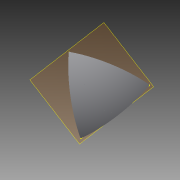
# Autodesk Inventor part: ommatid
Saved by Autodesk Inventor 2015 SP2 (Build 190223200, 223)
## iProperties
Created: 2015-05-04
Part Number: ommatid
Material: Generic
Document SubType Name: Modeling
Designer: foote
Density: 1 g/cm^3
Appearance: Default
Mass: 180.071 g
Surface Area: 758.025 cm^2
Volume: 180.071 cm^3
Author: foote
Autodesk Inventor part; units mm, degrees
note: some values were not read from the file. Chosen so that the rebuilt part matches the saved one: kept side of "Split8".
sketch "Sketch1" plane through (0, 0, 0) normal (0, 0, 1) x (1, 0, 0)
  line L0 (-46.99, -29.0414) -> (46.99, -29.0414)
  line L1 (46.99, -29.0414) -> (46.99, 29.0414)
  line L2 (46.99, 29.0414) -> (-46.99, 29.0414)
  line L3 (-46.99, 29.0414) -> (-46.99, -29.0414)
  point P0 (0, 0)
  dimension "d3" = 46.99
  dimension "d4" = 46.99
  dimension "d5" = 29.0414
  dimension "d6" = 29.0414
  constraints: 8 end point, 2 parallel, 1 horizontal, 1 perpendicular
  measures "d3" distance from line of point (0, 0) L3
  measures "d4" distance from line of L1 point (0, 0)
  measures "d5" distance from line of L0 point (0, 0)
  measures "d6" distance from line of L2 point (0, 0)
sketch "Sketch4" plane through (0, 0, 0) normal (1, 0, 0) x (0, 1, 0)
  line L0 (-47.0942, 0) -> (47.0942, 0)
  line L1 (-46.99, -29.0414) -> (46.99, -29.0414)
  line L2 (46.99, -29.0414) -> (46.99, 29.0414)
  line L3 (46.99, 29.0414) -> (-46.99, 29.0414)
  line L4 (-46.99, 29.0414) -> (-46.99, -29.0414)
  point P0 (0, 0)
  point P1 (0, 0)
  dimension "d38" = 29.0414
  dimension "d39" = 29.0414
  dimension "d40" = 46.99
  dimension "d41" = 46.99
  constraints: 10 end point, 2 parallel, 1 horizontal, 1 midpoint, 1 perpendicular
  measures "d38" distance from line of L3 point (0, 0)
  measures "d39" distance from line of L1 point (0, 0)
  measures "d40" distance from line of L2 point (0, 0)
  measures "d41" distance from line of L4 point (0, 0)
sketch "Sketch5" plane through (0, 0, 0) normal (0, 1, 0) x (-1, 0, 0)
  line L0 (-29.0414, -46.99) -> (29.0414, -46.99)
  line L1 (29.0414, -46.99) -> (29.0414, 46.99)
  line L2 (29.0414, 46.99) -> (-29.0414, 46.99)
  line L3 (-29.0414, 46.99) -> (-29.0414, -46.99)
  point P0 (0, 0)
  point P1 (0, 0)
  point P2 (0, 0)
  dimension "d31" = 29.0414
  dimension "d32" = 29.0414
  dimension "d33" = 46.99
  dimension "d34" = 46.99
  constraints: 8 end point, 2 parallel, 1 coincident, 1 horizontal, 1 perpendicular
  measures "d31" distance from line of point (0, 0) L3
  measures "d32" distance from line of L1 point (0, 0)
  measures "d33" distance from line of L0 point (0, 0)
  measures "d34" distance from line of L2 point (0, 0)
sketch3d "3D Sketch1"
ref_plane "Work Plane1" through (0, 46.99, 29.0414) normal (-0.5773503, -0.5773503, -0.5773503) x (0.809017, -0.309017, -0.5)
sketch "Sketch6" plane through (0, 46.99, 29.0414) normal (-0.5773503, -0.5773503, -0.5773503) x (0.809017, -0.309017, -0.5)
  line L0 (0, 0) -> (29.0414, 50.3012) projected
  line L1 (0, 0) -> (58.0828, 0) projected
  line L2 (29.0414, 50.3012) -> (58.0828, 0) projected
  line L3 (14.5207, 25.1506) -> (29.0414, 0)
  line L4 (29.0414, 0) -> (43.5621, 25.1506)
  line L5 (14.5207, 25.1506) -> (43.5621, 25.1506)
  circle A0 centre (29.0414, 16.7671) radius 12.7
  dimension "d48" = 25.4
  constraints: 6 end point, 3 midpoint, 1 centre point, 1 coincident, 1 horizontal
  measures "d48" diameter of A0
sketch3d "3D Sketch2"
ref_plane "Work Plane2" through (-6.7458, 40.2442, 22.2957) normal (-0.5773503, -0.5773503, -0.5773503) x (0.809017, -0.309017, -0.5)
sketch "Sketch8" plane through (-6.7458, 40.2442, 22.2957) normal (-0.5773503, -0.5773503, -0.5773503) x (0.809017, -0.309017, -0.5)
  line L0 (18.3857, 22.9192) -> (39.6971, 22.9192)
  line L1 (39.6971, 22.9192) -> (29.0414, 4.4629)
  line L2 (29.0414, 4.4629) -> (18.3857, 22.9192)
  line L3 (29.0414, 4.4629) -> (50.3529, 4.4629)
  line L4 (39.6971, 22.9192) -> (50.3529, 4.4629)
  line L5 (7.73, 4.4629) -> (18.3857, 22.9192)
  line L6 (7.73, 4.4629) -> (29.0414, 4.4629)
  line L7 (39.6971, 22.9192) -> (29.0414, 41.3754)
  line L8 (18.3857, 22.9192) -> (29.0414, 41.3754)
  point P0 (29.0414, 16.7671)
  constraints: 18 end point, 3 horizontal
ref_plane "Work Plane4" through (0, 46.99, 29.0414) normal (-0.809017, -0.309017, 0.5) x (0, -0.8506508, -0.5257311)
sketch "Sketch9" plane through (0, 46.99, 29.0414) normal (-0.809017, -0.309017, 0.5) x (0, -0.8506508, -0.5257311)
  line L0 (0, 0) -> (55.2401, 0) projected
  line L1 (55.2401, 0) -> (30.536, 49.4082) projected
  line L2 (0, 0) -> (14.7032, 0)
  line L3 (30.536, 49.4082) -> (37.1114, 36.2572)
  line L4 (55.2401, 0) -> (79.9442, 39.9721) construction
  arc A0 (30.536, 49.4082) -> (0, 0) centre (55.2401, 0) ccw
  dimension "d43" = 46.99
  constraints: 6 end point, 2 point on circle, 1 centre point, 1 coincident, 1 collinear, 1 horizontal
  measures "d43" distance of L0.end L4.end
ref_plane "Work Plane7" through (0, 46.99, 29.0414) normal (-0.309017, 0.5, -0.809017) x (0.809017, -0.309017, -0.5)
ref_plane "Work Plane9" through (46.99, 29.0414, 0) normal (-0.1624598, 0.2628656, 0.9510565) x (-0.8506508, -0.5257311, 0)
revolve "Revolution2" add sketch "Sketch9" angle 58.283 about axis through (0, 0, 0) along (-0.5, 0.809017, -0.309017)
ref_plane "Work Plane10" through (0, 0, 0) normal (0.5, -0.809017, -0.309017) x (0.8506508, 0.5257311, 0)
ref_plane "Work Plane11" through (0, 46.99, 29.0414) normal (-0.309017, 0.5, -0.809017) x (0.809017, -0.309017, -0.5)
split "Split4" plane through (0, 0, 0) removes the side toward (0.5, -0.809017, -0.309017)
split "Split5" plane through (0, 46.99, 29.0414) removes the side toward (-0.309017, 0.5, -0.809017)
ref_plane "Work Plane13" through (18.7929, 30.4076, 49.2006) normal (0, 0.8506508, -0.5257311) x (0.809017, -0.309017, -0.5)
ref_plane "Work Plane14" through (49.2006, 18.7929, 30.4076) normal (-0.5257311, 0, 0.8506508) x (-0.5, 0.809017, -0.309017)
ref_plane "Work Plane15" through (0, 0, 0) normal (-0.8506508, 0.5257311, 0) x (0.309017, 0.5, 0.809017)
split body "Split7" result two bodies by plane through (0, 0, 0) normal (-0.8506508, 0.5257311, 0) first body at (17.4067, 29.1157, 14.0495)
split body "Split8" result two bodies by plane through (49.2006, 18.7929, 30.4076) normal (-0.5257311, 0, 0.8506508) bodies 3 first body at (26.8909, 19.1826, 16.0317)
split body "Split9" result two bodies by plane through (18.7929, 30.4076, 49.2006) normal (0, 0.8506508, -0.5257311) bodies 5 first body at (26.3652, 19.1826, 16.8824)
shell "Shell1" [suppressed]
shell "Shell2" [suppressed]
split "Split10" plane through (-6.7458, 40.2442, 22.2957) removes the side toward (-0.5773503, -0.5773503, -0.5773503)
split "Split11" plane through (-6.7458, 40.2442, 22.2957) removes the side toward (-0.5773503, -0.5773503, -0.5773503)
split "Split12" plane through (-6.7458, 40.2442, 22.2957) removes the side toward (-0.5773503, -0.5773503, -0.5773503)
split "Split13" plane through (-6.7458, 40.2442, 22.2957) removes the side toward (-0.5773503, -0.5773503, -0.5773503)
ref_plane "Work Plane16" through (29.0414, 0, 46.99) normal (0.5773503, 0.5773503, 0.5773503) x (0.309017, 0.5, -0.809017)
sketch "Sketch17" plane through (29.0414, 0, 46.99) normal (0.5773503, 0.5773503, 0.5773503) x (0.309017, 0.5, -0.809017)
  point P0 (29.0414, 16.7671)
equation "\"d3\" = radius"
equation "\"d4\" = radius"
equation "\"d40\" = radius"
equation "\"d41\" = radius"
equation "\"d33\" = radius"
equation "\"d34\" = radius"
equation "\"d43\" = radius"
equation "\"d46\" = wall_thick"
equation "\"d47\" = wall_thick"
equation "\"radius\" = 46.99"
equation "\"inset\" = 11.684"
equation "\"gratio\" = 1.618034"
equation "\"d11\" = radius"
equation "\"d12\" = gratio"
equation "\"d17\" = radius"
equation "\"d18\" = gratio"
equation "\"d23\" = radius"
equation "\"d24\" = gratio"
equation "\"d29\" = radius"
equation "\"d30\" = gratio"
equation "\"d35\" = radius"
equation "\"d36\" = gratio"
equation "\"d37\" = inset"
equation "\"wall_thick\" = 1.27"
body "Solid2"
body "Solid4"
body "Solid6"
body "Solid7"
